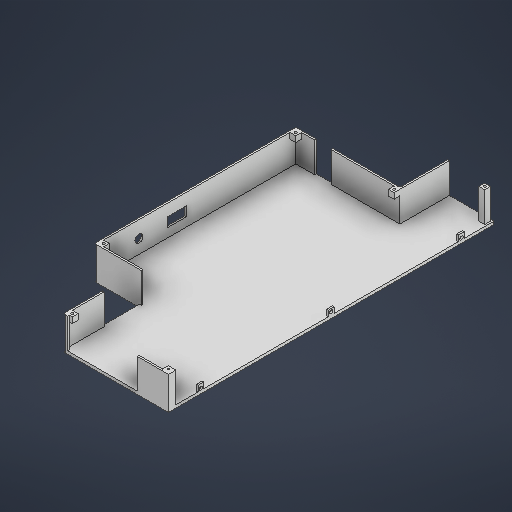
# Autodesk Inventor part: PCB_Grundplatte_Platinengehäuse_V2
Saved by Autodesk Inventor 2027 (Build 310192060, 192F)
## iProperties
Created: 2026-05-05
Part Number: PCB_Grundplatte_Platinengehäuse_V2
Material: Generisch
Document SubType Name: Modeling
Designer: simon
Density: 1 g/cm^3
Appearance: Vorgabe
Author: simon
Autodesk Inventor part; units mm, degrees
ref_plane "YZ Plane" through (0, 0, 0) normal (1, 0, 0) x (0, 1, 0)
ref_plane "XZ Plane" through (0, 0, 0) normal (0, 1, 0) x (-1, 0, 0)
ref_plane "XY Plane" through (0, 0, 0) normal (0, 0, 1) x (1, 0, 0)
sketch "Skizze1" plane through (0, 0, 0) normal (0, 0, 1) x (1, 0, 0)
  line L0 (-55, 75) -> (55, 75)
  line L1 (55, 75) -> (55, -75)
  line L2 (55, -75) -> (-55, -75) construction
  line L3 (-55, -75) -> (-55, 75)
  line L4 (0, -221.26) -> (0, 172.56) construction
  line L5 (-81, 0) -> (101, 0) construction
  line L6 (55, -75) -> (-16, -75) construction
  line L7 (-16, -75) -> (-16, -165) construction
  line L8 (-16, -165) -> (55, -165)
  line L9 (55, -165) -> (55, -75)
  line L10 (55, -165) -> (75, -165)
  line L11 (75, -165) -> (75, 116.3)
  line L12 (75, 116.3) -> (55, 116.3)
  line L13 (55, 116.3) -> (55, -165) construction
  line L14 (-55, -75) -> (-16, -75) construction
  line L15 (-16, -75) -> (-16, -99) construction
  line L16 (-16, -99) -> (-55, -99)
  line L17 (-55, -99) -> (-55, -75)
  line L18 (-16, -99) -> (-16, -165)
  line L19 (55, 116.3) -> (35, 116.3)
  line L20 (35, 116.3) -> (35, 75)
  line L21 (35, 75) -> (55, 75)
  line L22 (55, 75) -> (55, 116.3) construction
  point P0 (0, 0)
  point P1 (-35.5, -75)
  dimension "d0" = 110
  dimension "d1" = 150
  dimension "d4" = 90
  dimension "d5" = 71
  dimension "d6" = 281.3
  dimension "d7" = 20
  dimension "d139" = 24
  dimension "d140" = 20
  constraints: 42 end point, 10 parallel, 6 perpendicular, 5 horizontal, 2 point on line, 1 midpoint, 2 other
  measures "d0" distance of L0.start L0.end
  measures "d1" distance between parallel lines of L0 L2
  measures "d4" distance of L8.end L1.end
  measures "d5" distance of L7.end L8.end
  measures "d6" distance between parallel lines of L10 L12
  measures "d7" distance of L11.end L12.end
  measures "d139" distance from line of point (-35.5, -75) L16
  measures "d140" distance between parallel lines of L22 L20
extrude "Extrusion1" add sketch "Skizze1" along normal blind 2.5
sketch "Skizze7" plane through (0, 0, 2.5) normal (0, 0, 1) x (1, 0, 0)
  line L0 (75, 116.3) -> (35, 116.3) projected
  line L1 (75, 116.3) -> (73.5, 116.3)
  line L2 (73.5, 116.3) -> (73.5, -165) construction
  line L3 (73.5, -165) -> (75, -165)
  line L4 (75, -165) -> (75, 116.3)
  line L5 (75, 90.67) -> (73.5, 90.67)
  line L6 (73.5, 90.67) -> (73.5, 85.67)
  line L7 (73.5, 85.67) -> (75, 85.67)
  line L8 (75, 85.67) -> (75, 90.67)
  line L9 (75, -134.37) -> (73.5, -134.37)
  line L10 (73.5, -134.37) -> (73.5, -139.37)
  line L11 (73.5, -139.37) -> (75, -139.37)
  line L12 (75, -139.37) -> (75, -134.37)
  line L13 (-16, -165) -> (75, -165) projected
  line L14 (75, -165) -> (75, 116.3) projected
  line L15 (75, -26.85) -> (73.5, -26.85)
  line L16 (73.5, -26.85) -> (73.5, -21.85)
  line L17 (73.5, -21.85) -> (75, -21.85)
  line L18 (75, -21.85) -> (75, -26.85)
  point P0 (0, 0)
  point P1 (45.75, 136.3)
  point P2 (-15.25, -145)
  point P3 (75, 85.67)
  point P4 (49.25, 116.3)
  point P5 (74.25, -165)
  point P6 (75, -26.85)
  point P7 (75, -21.85)
  dimension "d66" = 1.5
  dimension "d67" = 5
  dimension "d68" = 25.63
  dimension "d69" = 25.63
  dimension "d70" = 5
  dimension "d156" = 5
  dimension "d157" = 138.15
  constraints: 32 end point, 8 parallel, 7 point on line, 4 horizontal, 4 perpendicular, 1 midpoint, 1 other
  measures "d66" distance between parallel lines of L4 L2
  measures "d67" distance between parallel lines of L7 L5
  measures "d69" distance between parallel lines of L3 L11
  measures "d70" distance between parallel lines of L11 L9
  measures "d156" distance of L15.end L16.end
  measures "d157" distance between parallel lines of L15 L13
extrude "Extrusion6" add sketch "Skizze7" along normal blind 5
sketch "Skizze8" plane through (73.5, -139.37, 2.5) normal (-1, 0, 0) x (0, 0, 1)
  line L0 (0, 0) -> (5, 0) projected
  line L1 (5, 5) -> (5, 0) projected
  line L2 (0, 225.04) -> (5, 225.04) projected
  line L3 (5, 230.04) -> (5, 225.04) projected
  line L4 (0, 230.04) -> (5, 230.04) projected
  line L5 (0, 225.04) -> (0, 230.04) projected
  line L6 (5, 112.52) -> (5, 117.52) projected
  line L7 (0, 112.52) -> (5, 112.52) projected
  point P0 (-2.5, 139.37)
  point P1 (1.5, 2.5)
  point P2 (2.5, 0)
  point P3 (1.5, 227.54)
  point P4 (2.5, 115.02)
  dimension "d73" = 2.5
  dimension "d74" = 3.5
  dimension "d75" = 3.5
  dimension "d76" = 2.5
  dimension "d158" = 2.5
  dimension "d159" = 2.5
  constraints: 1 midpoint
  measures "d73" vertical distance of point (2.5, 0) point (1.5, 2.5)
  measures "d74" distance from line of L1 point (1.5, 2.5)
  measures "d75" distance from line of L3 point (1.5, 227.54)
  measures "d76" distance from line of L2 point (1.5, 227.54)
  measures "d158" distance from line of L6 point (2.5, 115.02)
  measures "d159" distance from line of L7 point (2.5, 115.02)
hole "Bohrung1" at (73.5, 88.17, 4) at (73.5, -136.87, 4) at (73.5, -24.35, 5) direction (1, 0, 0) diameter 3 depth 1.5
sketch "Skizze15" plane through (0, 0, 2.5) normal (0, 0, 1) x (1, 0, 0)
  line L0 (73.5, -134.37) -> (75, -134.37) projected
  line L1 (75, -134.37) -> (75, -26.85) projected
  line L2 (75, 85.67) -> (73.5, 85.67) projected
  line L3 (73.5, 85.67) -> (73.5, 88.17) projected
  line L4 (73.5, 88.17) -> (73.5, 90.67) projected
  line L5 (73.5, 90.67) -> (75, 90.67) projected
  line L6 (75, 90.67) -> (75, 116.3) projected
  line L7 (75, 116.3) -> (35, 116.3) projected
  line L8 (35, 116.3) -> (35, 75) projected
  line L9 (35, 75) -> (-55, 75) projected
  line L10 (-55, 75) -> (-55, -99) projected
  line L11 (-55, -99) -> (-16, -99) projected
  line L12 (-16, -99) -> (-16, -165) projected
  line L13 (-16, -165) -> (75, -165) projected
  line L14 (75, -165) -> (75, -139.37) projected
  line L15 (75, -139.37) -> (73.5, -139.37) projected
  line L16 (73.5, -139.37) -> (73.5, -136.87) projected
  line L17 (73.5, -136.87) -> (73.5, -134.37) projected
  line L18 (75, 116.3) -> (35, 116.3) projected
  line L19 (36.5, 116.3) -> (36.5, 73.5)
  line L20 (36.5, 73.5) -> (-23, 73.5)
  line L21 (-23, 73.5) -> (-23, 75)
  line L22 (-37, 75) -> (-37, 73.5)
  line L23 (-37, 73.5) -> (-53.5, 73.5)
  line L24 (-53.5, 73.5) -> (-53.5, -97.5)
  line L25 (-53.5, -97.5) -> (-14.5, -97.5)
  line L26 (-14.5, -97.5) -> (-14.5, -99)
  line L27 (-14.5, -99) -> (-16, -99)
  line L28 (-14.5, -131) -> (-14.5, -163.5)
  line L29 (-14.5, -163.5) -> (-12, -163.5)
  line L30 (-12, -163.5) -> (-12, -165)
  line L31 (48, -165) -> (48, -163.5)
  line L32 (48, -163.5) -> (75, -163.5)
  line L33 (-14.5, -131) -> (-16, -131)
  line L34 (75, -26.85) -> (73.5, -26.85) projected
  line L35 (73.5, -26.85) -> (73.5, -21.85) projected
  line L36 (73.5, -21.85) -> (75, -21.85) projected
  line L37 (75, -21.85) -> (75, 85.67) projected
  line L38 (75, 111.3) -> (75, 116.3)
  line L39 (75, -163.5) -> (73.5, -163.5)
  line L40 (73.5, -163.5) -> (73.5, -158.5)
  line L41 (73.5, -158.5) -> (75, -158.5)
  line L42 (75, -158.5) -> (75, -163.5)
  line L43 (73.5, 114.8) -> (68.5, 114.8)
  line L44 (68.5, 114.8) -> (68.5, 109.8)
  line L45 (68.5, 109.8) -> (73.5, 109.8)
  line L46 (73.5, 109.8) -> (73.5, 114.8)
  point P0 (0, 0)
  point P1 (75, -158.5)
  dimension "d141" = 1.5
  dimension "d142" = 1.5
  dimension "d143" = 1.5
  dimension "d144" = 1.5
  dimension "d145" = 1.5
  dimension "d146" = 1.5
  dimension "d147" = 4
  dimension "d148" = 64
  dimension "d149" = 0
  dimension "d150" = 32
  dimension "d151" = 18
  dimension "d152" = 14
  dimension "d171" = 5
  dimension "d172" = 1.5
  dimension "d224" = 5
  dimension "d225" = 5
  dimension "d226" = 1.5
  dimension "d227" = 1.5
  constraints: 48 end point, 14 point on line, 13 perpendicular, 5 parallel, 2 horizontal
  measures "d141" distance between parallel lines of L9 L20
  measures "d142" distance between parallel lines of L8 L19
  measures "d143" distance between parallel lines of L10 L24
  measures "d144" distance between parallel lines of L11 L25
  measures "d145" distance between parallel lines of L12 L26
  measures "d146" distance between parallel lines of L13 L29
  measures "d147" distance between parallel lines of L12 L30
  measures "d148" distance between parallel lines of L12 L31
  measures "d149" distance from line of L11 L26.end
  measures "d150" distance from line of L33 L26.end
  measures "d151" distance between parallel lines of L10 L22
  measures "d152" distance between parallel lines of L21 L22
  measures "d171" distance of L39.end L40.end
  measures "d172" distance between parallel lines of L42 L40
  measures "d224" distance of L45.end L44.end
  measures "d225" distance of L44.end L43.end
  measures "d226" distance between parallel lines of L7 L43
  measures "d227" distance between parallel lines of L6 L46
extrude "Extrusion13" add sketch "Skizze15" along normal blind 26 contours L14 L32 L40 L41 | L14 L13 L31 L32 | L13 L12 L33 L28 L29 L30 | L11 L10 L9 L22 L23 L24 L25 L26 L27 | L19 L20 L21 L9 L8 L7 | L46 L45 L44 L43
fillet "Rundung1" radius 2 4 edges at (35, 75, 14.25) (-55, 75, 14.25) (-55, -99, 14.25) (-16, -165, 14.25)
sketch "Skizze16" plane through (-55, -97, 0) normal (-1, 0, 0) x (0, 0, 1)
  line L0 (18.35, 76.1) -> (10.15, 76.1)
  line L1 (10.15, 76.1) -> (10.15, 60)
  line L2 (10.15, 60) -> (18.35, 60)
  line L3 (18.35, 60) -> (18.35, 76.1)
  circle A0 centre (14.25, 35) radius 3.5
  line L4 (0, 170) -> (28.5, 170) projected
  line L5 (0, 170) -> (0, 0) projected
  line L6 (28.5, 0) -> (0, 0) projected
  line L7 (28.5, 170) -> (28.5, 0) projected
  point P0 (0, 97)
  dimension "d160" = 16.1
  dimension "d161" = 8.2
  dimension "d162" = 7
  dimension "d163" = 14.25
  dimension "d164" = 35
  dimension "d165" = 60
  dimension "d166" = 10.15
  constraints: 8 end point, 2 parallel, 1 centre point, 1 horizontal, 1 perpendicular
  measures "d160" distance of L1.end L0.end
  measures "d161" distance of L1.end L2.end
  measures "d162" diameter of A0
  measures "d163" distance from line of L5 A0.centre
  measures "d164" distance from line of L6 A0.centre
  measures "d165" distance between parallel lines of L2 L6
  measures "d166" distance between parallel lines of L5 L1
extrude "Extrusion14" cut sketch "Skizze16" against normal up to surface (1.5 mm away) contours L3 L2 L1 L0 | A0
sketch "Skizze17" plane through (0, 0, 28.5) normal (0, 0, 1) x (1, 0, 0)
  line L0 (73.5, -163.5) -> (48, -163.5) projected
  line L1 (73.5, -163.5) -> (68.5, -163.5)
  line L2 (68.5, -163.5) -> (68.5, -158.5)
  line L3 (68.5, -158.5) -> (73.5, -158.5)
  line L4 (73.5, -158.5) -> (73.5, -163.5)
  line L5 (-14.5, -131) -> (-14.5, -163.5) projected
  line L6 (-14.5, -163.5) -> (-9.5, -163.5)
  line L7 (-9.5, -163.5) -> (-9.5, -158.5)
  line L8 (-9.5, -158.5) -> (-14.5, -158.5)
  line L9 (-14.5, -158.5) -> (-14.5, -163.5)
  line L10 (-53.5, 73.5) -> (-53.5, -97.5) projected
  line L11 (-53.5, -97.5) -> (-48.5, -97.5)
  line L12 (-48.5, -97.5) -> (-48.5, -92.5)
  line L13 (-48.5, -92.5) -> (-53.5, -92.5)
  line L14 (-53.5, -92.5) -> (-53.5, -97.5)
  line L15 (-53.5, 73.5) -> (-48.5, 73.5)
  line L16 (-48.5, 73.5) -> (-48.5, 68.5)
  line L17 (-48.5, 68.5) -> (-53.5, 68.5)
  line L18 (-53.5, 68.5) -> (-53.5, 73.5)
  line L19 (36.5, 73.5) -> (36.5, 116.3) projected
  line L20 (36.5, 73.5) -> (31.5, 73.5)
  line L21 (31.5, 73.5) -> (31.5, 68.5)
  line L22 (31.5, 68.5) -> (36.5, 68.5)
  line L23 (36.5, 68.5) -> (36.5, 73.5)
  point P0 (0, 0)
  point P1 (-14.5, -158.5)
  dimension "d173" = 5
  dimension "d174" = 5
  dimension "d175" = 5
  dimension "d176" = 5
  dimension "d177" = 5
  dimension "d178" = 5
  dimension "d179" = 5
  dimension "d180" = 5
  dimension "d181" = 5
  dimension "d182" = 5
  constraints: 40 end point, 10 parallel, 5 horizontal, 5 perpendicular
  measures "d173" distance of L2.end L3.end
  measures "d174" distance of L1.end L2.end
  measures "d175" distance of L8.end L7.end
  measures "d176" distance of L7.end L6.end
  measures "d177" distance of L13.end L12.end
  measures "d178" distance of L12.end L11.end
  measures "d179" distance of L16.end L17.end
  measures "d180" distance of L15.end L16.end
  measures "d181" distance of L22.end L21.end
  measures "d182" distance of L21.end L20.end
extrude "Extrusion15" add sketch "Skizze17" against normal blind 5
sketch "Skizze19" plane through (0, 0, 28.5) normal (0, 0, 1) x (1, 0, 0)
  line L0 (-14, -165) -> (75, -165) projected
  line L1 (75, -165) -> (75, -158.5) projected
  line L2 (-12, -165) -> (48, -165) projected
  line L3 (-16, -131) -> (-16, -163) projected
  line L4 (-53, -99) -> (-14.5, -99) projected
  line L5 (-55, 73) -> (-55, -97) projected
  line L6 (33, 75) -> (-53, 75) projected
  line L7 (33, 75) -> (-53, 75) projected
  line L8 (31.5, 73.5) -> (31.5, 68.5) projected
  line L9 (36.5, 116.3) -> (35, 116.3) projected
  line L10 (75, 90.67) -> (75, 116.3) projected
  point P0 (0, 0)
  point P1 (71, -161)
  point P2 (-12, -161)
  point P3 (-51, -95)
  point P4 (-51, 71)
  point P5 (34, 71)
  point P6 (71, 112.3)
  point P7 (-16, -163)
  point P8 (-37, 75)
  point P9 (-23, 75)
  point P10 (69.25, -139.37)
  point P11 (-21.75, -99)
  dimension "d205" = 4
  dimension "d206" = 4
  dimension "d207" = 4
  dimension "d208" = 4
  dimension "d209" = 4
  dimension "d210" = 4
  dimension "d211" = 4
  dimension "d212" = 4
  dimension "d213" = 4
  dimension "d214" = 2.5
  dimension "d215" = 4
  dimension "d228" = 4
  constraints: 2 other
  measures "d205" distance from line of point (71, -161) L0
  measures "d207" distance from line of L2 point (-12, -161)
  measures "d209" distance from line of L4 point (-51, -95)
  measures "d210" distance from line of L5 point (-51, -95)
  measures "d211" distance from line of L5 point (-51, 71)
  measures "d212" distance from line of L6 point (-51, 71)
  measures "d213" distance from line of L7 point (34, 71)
  measures "d214" distance from line of L8 point (34, 71)
  measures "d215" distance from line of L9 point (71, 112.3)
  measures "d228" distance from line of L10 point (71, 112.3)
hole "Bohrung3" at (71, -161, 28.5) at (-12, -161, 28.5) at (-51, -95, 28.5) at (71, 112.3, 28.5) at (34, 71, 28.5) at (-51, 71, 28.5) direction (0, 0, -1) diameter 2 depth 5
